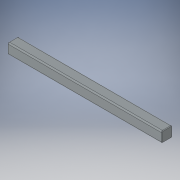
# Autodesk Inventor part: Axle 5s
Saved by Autodesk Inventor 2019 (Build 230136000, 136)
## iProperties
Company: Unknown
Created: 2018-11-05
Part Number: Axle 5s
Material: Generic
Description: Unknown
Document SubType Name: Modeling
Designer: Varga Daniel
Density: 1 g/cm^3
Appearance: Default
Title: Axeis 5s
Author: Unknown
Autodesk Inventor part; units mm, degrees
ref_plane "YZ Plane" through (0, 0, 0) normal (1, 0, 0) x (0, 1, 0)
ref_plane "XZ Plane" through (0, 0, 0) normal (0, 1, 0) x (-1, 0, 0)
ref_plane "XY Plane" through (0, 0, 0) normal (0, 0, 1) x (1, 0, 0)
feature "Base1" [suppressed]
thicken "Thicken1" [suppressed]
ref_plane "Work Plane1" through (-1.4, -18.2, -1.4) normal (-0.7071, 0, 0.7071) x (0.7071, 0, 0.7071)
ref_plane "Work Plane2" through (1.5414, 21.8, -1.5414) normal (-0.7071, 0, 0.7071) x (0, -1, 0)
ref_plane "Work Plane3" through (-1.5414, 21.8, 1.5414) normal (-0.7071, 0, 0.7071) x (0, -1, 0)
sketch "Sketch1" plane through (0, 0, 0) normal (1, 0, 0) x (0, 1, 0)
  line L0 (1.325, 1.725) -> (-1.325, 1.725)
  line L1 (-1.725, 1.325) -> (-1.725, -1.325)
  line L2 (-1.325, -1.725) -> (1.325, -1.725)
  line L3 (1.725, -1.325) -> (1.725, 1.325)
  line L4 (1.725, 1.725) -> (-1.725, -1.725) construction
  line L5 (-1.725, 1.725) -> (1.725, -1.725) construction
  arc A0 (1.725, 1.325) -> (1.325, 1.725) centre (1.325, 1.325) ccw
  arc A1 (-1.325, 1.725) -> (-1.725, 1.325) centre (-1.325, 1.325) ccw
  arc A2 (-1.725, -1.325) -> (-1.325, -1.725) centre (-1.325, -1.325) ccw
  arc A3 (1.325, -1.725) -> (1.725, -1.325) centre (1.325, -1.325) ccw
  point P0 (0, 0)
  dimension "d2" = 3.45
  dimension "d3" = 3.45
  dimension "d4" = 0.4
  constraints: 12 end point, 8 point on circle, 8 point on line, 8 tangent, 4 centre point, 3 equal radius, 2 midpoint, 2 parallel, 1 horizontal, 1 perpendicular
  measures "d2" distance of L5.end L4.end
  measures "d3" distance between parallel lines of L0 L2
  measures "d4" radius of A0
extrude "Extrusion1" add sketch "Sketch1" along normal blind 50
fillet "Fillet1" radius 0.2 16 edges at (50, 1.6078, 1.6078) (50, 0, 1.725) (50, -1.6078, 1.6078) (50, -1.725, 0) (50, -1.6078, -1.6078) (50, 0, -1.725) (50, 1.6078, -1.6078) (50, 1.725, 0) (0, 1.6078, 1.6078) (0, 0, 1.725) (0, -1.6078, 1.6078) (0, -1.725, 0) (0, -1.6078, -1.6078) (0, 0, -1.725) (0, 1.6078, -1.6078) (0, 1.725, 0)
equation "\"d3\" = d2"
body "Solid1"
